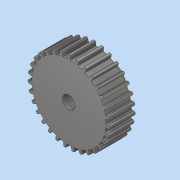
# Autodesk Inventor part: PinionGear
Saved by Autodesk Inventor 2017 (Build 210142000, 142)
## iProperties
Created: 2016-11-06
Part Number: PinionGear
Material: Stainless Steel, Brushed
Document SubType Name: Modeling
Designer: techn
Density: 8 g/cm^3
Appearance: Stainless - Brushed
Author: techn
Comments: 31 Tooth Traxxas Pinion Gear
Autodesk Inventor part; units mm, degrees
ref_plane "YZ Plane" through (0, 0, 0) normal (1, 0, 0) x (0, 1, 0)
ref_plane "XZ Plane" through (0, 0, 0) normal (0, 1, 0) x (-1, 0, 0)
ref_plane "XY Plane" through (0, 0, 0) normal (0, 0, 1) x (1, 0, 0)
sketch "Sketch1" plane through (0, 0, 0) normal (0, 0, 1) x (1, 0, 0)
  circle A0 centre (0, 0) radius 3.7465
  dimension "d0" = 7.493
  constraints: 1 centre point, 1 coincident
  measures "d0" diameter of A0
extrude "Extrusion1" add sketch "Sketch1" along normal blind 10.5156
sketch "Sketch2" plane through (0, 0, 10.5156) normal (0, 0, 1) x (1, 0, 0)
  circle A0 centre (0, 0) radius 10.16
  dimension "d3" = 20.32
  constraints: 1 centre point, 1 coincident
  measures "d3" diameter of A0
extrude "Extrusion2" add sketch "Sketch2" against normal blind 6.35
sketch "Sketch4" plane through (0, 0, 10.5156) normal (0, 0, 1) x (1, 0, 0)
  circle A0 centre (0, 0) radius 1.5875
  dimension "d6" = 3.175
  constraints: 1 centre point, 1 coincident
  measures "d6" diameter of A0
extrude "Extrusion3" cut sketch "Sketch4" against normal through all
sketch "Sketch5" plane through (0, 0, 10.5156) normal (0, 0, 1) x (1, 0, 0)
  circle A0 centre (0, 0) radius 9.2075
  line L0 (0.3683, 9.2001) -> (0.3683, 9.7081)
  line L1 (0.3683, 9.7081) -> (0.2667, 10.16)
  line L2 (0.2667, 10.16) -> (-0.2667, 10.16)
  line L3 (-0.2667, 10.16) -> (-0.3683, 9.7081)
  line L4 (-0.3683, 9.7081) -> (-0.3683, 9.2001)
  line L5 (-0.3683, 9.2001) -> (0.3683, 9.2001)
  line L6 (-2.315, 9.4353) -> (-2.2127, 8.9377)
  line L7 (-2.3064, 9.8983) -> (-2.315, 9.4353)
  line L8 (-1.784, 10.0057) -> (-2.3064, 9.8983)
  line L9 (-1.5935, 9.5835) -> (-1.784, 10.0057)
  line L10 (-1.4912, 9.0859) -> (-1.5935, 9.5835)
  line L11 (-2.2127, 8.9377) -> (-1.4912, 9.0859)
  line L12 (-4.1669, 8.7761) -> (-3.9666, 8.3093)
  line L13 (-4.2517, 9.2314) -> (-4.1669, 8.7761)
  line L14 (-3.7616, 9.4418) -> (-4.2517, 9.2314)
  line L15 (-3.49, 9.0666) -> (-3.7616, 9.4418)
  line L16 (-3.2897, 8.5998) -> (-3.49, 9.0666)
  line L17 (-3.9666, 8.3093) -> (-3.2897, 8.5998)
  line L18 (-5.8482, 7.7577) -> (-5.558, 7.3407)
  line L19 (-6.023, 8.1866) -> (-5.8482, 7.7577)
  line L20 (-5.5852, 8.4913) -> (-6.023, 8.1866)
  line L21 (-5.2437, 8.1785) -> (-5.5852, 8.4913)
  line L22 (-4.9535, 7.7615) -> (-5.2437, 8.1785)
  line L23 (-5.558, 7.3407) -> (-4.9535, 7.7615)
  line L24 (-7.2901, 6.4216) -> (-6.9219, 6.0716)
  line L25 (-7.5476, 6.8066) -> (-7.2901, 6.4216)
  line L26 (-7.1801, 7.1932) -> (-7.5476, 6.8066)
  line L27 (-6.7826, 6.9555) -> (-7.1801, 7.1932)
  line L28 (-6.4144, 6.6055) -> (-6.7826, 6.9555)
  line L29 (-6.9219, 6.0716) -> (-6.4144, 6.6055)
  line L30 (-8.4336, 4.8227) -> (-8.0025, 4.554)
  line L31 (-8.7633, 5.1479) -> (-8.4336, 4.8227)
  line L32 (-8.4812, 5.6006) -> (-8.7633, 5.1479)
  line L33 (-8.0439, 5.4478) -> (-8.4812, 5.6006)
  line L34 (-7.6128, 5.1791) -> (-8.0439, 5.4478)
  line L35 (-8.0025, 4.554) -> (-7.6128, 5.1791)
  line L36 (-9.2317, 3.0263) -> (-8.7554, 2.8499)
  line L37 (-9.6202, 3.2785) -> (-9.2317, 3.0263)
  line L38 (-9.4349, 3.7787) -> (-9.6202, 3.2785)
  line L39 (-8.9759, 3.7171) -> (-9.4349, 3.7787)
  line L40 (-8.4995, 3.5406) -> (-8.9759, 3.7171)
  line L41 (-8.7554, 2.8499) -> (-8.4995, 3.5406)
  line L42 (-9.652, 1.106) -> (-9.1498, 1.0291)
  line L43 (-10.0832, 1.2749) -> (-9.652, 1.106)
  line L44 (-10.0025, 1.8021) -> (-10.0832, 1.2749)
  line L45 (-9.5404, 1.8341) -> (-10.0025, 1.8021)
  line L46 (-9.0383, 1.7572) -> (-9.5404, 1.8341)
  line L47 (-9.1498, 1.0291) -> (-9.0383, 1.7572)
  line L48 (-9.677, -0.8595) -> (-9.1697, -0.8338)
  line L49 (-10.1335, -0.781) -> (-9.677, -0.8595)
  line L50 (-10.1605, -0.2482) -> (-10.1335, -0.781)
  line L51 (-9.7143, -0.1239) -> (-10.1605, -0.2482)
  line L52 (-9.207, -0.0982) -> (-9.7143, -0.1239)
  line L53 (-9.1697, -0.8338) -> (-9.207, -0.0982)
  line L54 (-9.3059, -2.7899) -> (-8.8141, -2.6626)
  line L55 (-9.7688, -2.8048) -> (-9.3059, -2.7899)
  line L56 (-9.9025, -2.2884) -> (-9.7688, -2.8048)
  line L57 (-9.4905, -2.0768) -> (-9.9025, -2.2884)
  line L58 (-8.9988, -1.9495) -> (-9.4905, -2.0768)
  line L59 (-8.8141, -2.6626) -> (-8.9988, -1.9495)
  line L60 (-8.5538, -4.6061) -> (-8.0977, -4.3823)
  line L61 (-9.0042, -4.7138) -> (-8.5538, -4.6061)
  line L62 (-9.2391, -4.235) -> (-9.0042, -4.7138)
  line L63 (-8.8782, -3.9447) -> (-9.2391, -4.235)
  line L64 (-8.4221, -3.721) -> (-8.8782, -3.9447)
  line L65 (-8.0977, -4.3823) -> (-8.4221, -3.721)
  line L66 (-7.4515, -6.2336) -> (-7.0498, -5.9227)
  line L67 (-7.871, -6.4299) -> (-7.4515, -6.2336)
  line L68 (-8.1975, -6.0081) -> (-7.871, -6.4299)
  line L69 (-7.9024, -5.6512) -> (-8.1975, -6.0081)
  line L70 (-7.5007, -5.3402) -> (-7.9024, -5.6512)
  line L71 (-7.0498, -5.9227) -> (-7.5007, -5.3402)
  line L72 (-6.0442, -7.606) -> (-5.7133, -7.2206)
  line L73 (-6.4156, -7.8827) -> (-6.0442, -7.606)
  line L74 (-6.8203, -7.5353) -> (-6.4156, -7.8827)
  line L75 (-6.6031, -7.1262) -> (-6.8203, -7.5353)
  line L76 (-6.2722, -6.7408) -> (-6.6031, -7.1262)
  line L77 (-5.7133, -7.2206) -> (-6.2722, -6.7408)
  line L78 (-4.3894, -8.667) -> (-4.1428, -8.2228)
  line L79 (-4.6975, -9.0128) -> (-4.3894, -8.667)
  line L80 (-5.1639, -8.7539) -> (-4.6975, -9.0128)
  line L81 (-5.0334, -8.3095) -> (-5.1639, -8.7539)
  line L82 (-4.7869, -7.8654) -> (-5.0334, -8.3095)
  line L83 (-4.1428, -8.2228) -> (-4.7869, -7.8654)
  line L84 (-2.5548, -9.3732) -> (-2.4028, -8.8885)
  line L85 (-2.7871, -9.7739) -> (-2.5548, -9.3732)
  line L86 (-3.296, -9.6142) -> (-2.7871, -9.7739)
  line L87 (-3.2577, -9.1527) -> (-3.296, -9.6142)
  line L88 (-3.1056, -8.668) -> (-3.2577, -9.1527)
  line L89 (-2.4028, -8.8885) -> (-3.1056, -8.668)
  line L90 (-0.6157, -9.6956) -> (-0.5644, -9.1902)
  line L91 (-0.7625, -10.1349) -> (-0.6157, -9.6956)
  line L92 (-1.2932, -10.0809) -> (-0.7625, -10.1349)
  line L93 (-1.3486, -9.6211) -> (-1.2932, -10.0809)
  line L94 (-1.2972, -9.1157) -> (-1.3486, -9.6211)
  line L95 (-0.5644, -9.1902) -> (-1.2972, -9.1157)
  line L96 (1.3486, -9.6211) -> (1.2972, -9.1157)
  line L97 (1.2932, -10.0809) -> (1.3486, -9.6211)
  line L98 (0.7625, -10.1349) -> (1.2932, -10.0809)
  line L99 (0.6157, -9.6956) -> (0.7625, -10.1349)
  line L100 (0.5644, -9.1902) -> (0.6157, -9.6956)
  line L101 (1.2972, -9.1157) -> (0.5644, -9.1902)
  line L102 (3.2577, -9.1527) -> (3.1056, -8.668)
  line L103 (3.296, -9.6142) -> (3.2577, -9.1527)
  line L104 (2.7871, -9.7739) -> (3.296, -9.6142)
  line L105 (2.5548, -9.3732) -> (2.7871, -9.7739)
  line L106 (2.4028, -8.8885) -> (2.5548, -9.3732)
  line L107 (3.1056, -8.668) -> (2.4028, -8.8885)
  line L108 (5.0334, -8.3095) -> (4.7869, -7.8654)
  line L109 (5.1639, -8.7539) -> (5.0334, -8.3095)
  line L110 (4.6975, -9.0128) -> (5.1639, -8.7539)
  line L111 (4.3894, -8.667) -> (4.6975, -9.0128)
  line L112 (4.1428, -8.2228) -> (4.3894, -8.667)
  line L113 (4.7869, -7.8654) -> (4.1428, -8.2228)
  line L114 (6.6031, -7.1262) -> (6.2722, -6.7408)
  line L115 (6.8203, -7.5353) -> (6.6031, -7.1262)
  line L116 (6.4156, -7.8827) -> (6.8203, -7.5353)
  line L117 (6.0442, -7.606) -> (6.4156, -7.8827)
  line L118 (5.7133, -7.2206) -> (6.0442, -7.606)
  line L119 (6.2722, -6.7408) -> (5.7133, -7.2206)
  line L120 (7.9024, -5.6512) -> (7.5007, -5.3402)
  line L121 (8.1975, -6.0081) -> (7.9024, -5.6512)
  line L122 (7.871, -6.4299) -> (8.1975, -6.0081)
  line L123 (7.4515, -6.2336) -> (7.871, -6.4299)
  line L124 (7.0498, -5.9227) -> (7.4515, -6.2336)
  line L125 (7.5007, -5.3402) -> (7.0498, -5.9227)
  line L126 (8.8782, -3.9447) -> (8.4221, -3.721)
  line L127 (9.2391, -4.235) -> (8.8782, -3.9447)
  line L128 (9.0042, -4.7138) -> (9.2391, -4.235)
  line L129 (8.5538, -4.6061) -> (9.0042, -4.7138)
  line L130 (8.0977, -4.3823) -> (8.5538, -4.6061)
  line L131 (8.4221, -3.721) -> (8.0977, -4.3823)
  line L132 (9.4905, -2.0768) -> (8.9988, -1.9495)
  line L133 (9.9025, -2.2884) -> (9.4905, -2.0768)
  line L134 (9.7688, -2.8048) -> (9.9025, -2.2884)
  line L135 (9.3059, -2.7899) -> (9.7688, -2.8048)
  line L136 (8.8141, -2.6626) -> (9.3059, -2.7899)
  line L137 (8.9988, -1.9495) -> (8.8141, -2.6626)
  line L138 (9.7143, -0.1239) -> (9.207, -0.0982)
  line L139 (10.1605, -0.2482) -> (9.7143, -0.1239)
  line L140 (10.1335, -0.781) -> (10.1605, -0.2482)
  line L141 (9.677, -0.8595) -> (10.1335, -0.781)
  line L142 (9.1697, -0.8338) -> (9.677, -0.8595)
  line L143 (9.207, -0.0982) -> (9.1697, -0.8338)
  line L144 (9.5404, 1.8341) -> (9.0383, 1.7572)
  line L145 (10.0025, 1.8021) -> (9.5404, 1.8341)
  line L146 (10.0832, 1.2749) -> (10.0025, 1.8021)
  line L147 (9.652, 1.106) -> (10.0832, 1.2749)
  line L148 (9.1498, 1.0291) -> (9.652, 1.106)
  line L149 (9.0383, 1.7572) -> (9.1498, 1.0291)
  line L150 (8.9759, 3.7171) -> (8.4995, 3.5406)
  line L151 (9.4349, 3.7787) -> (8.9759, 3.7171)
  line L152 (9.6202, 3.2785) -> (9.4349, 3.7787)
  line L153 (9.2317, 3.0263) -> (9.6202, 3.2785)
  line L154 (8.7554, 2.8499) -> (9.2317, 3.0263)
  line L155 (8.4995, 3.5406) -> (8.7554, 2.8499)
  line L156 (8.0439, 5.4478) -> (7.6128, 5.1791)
  line L157 (8.4812, 5.6006) -> (8.0439, 5.4478)
  line L158 (8.7633, 5.1479) -> (8.4812, 5.6006)
  line L159 (8.4336, 4.8227) -> (8.7633, 5.1479)
  line L160 (8.0025, 4.554) -> (8.4336, 4.8227)
  line L161 (7.6128, 5.1791) -> (8.0025, 4.554)
  line L162 (6.7826, 6.9555) -> (6.4144, 6.6055)
  line L163 (7.1801, 7.1932) -> (6.7826, 6.9555)
  line L164 (7.5476, 6.8066) -> (7.1801, 7.1932)
  line L165 (7.2901, 6.4216) -> (7.5476, 6.8066)
  line L166 (6.9219, 6.0716) -> (7.2901, 6.4216)
  line L167 (6.4144, 6.6055) -> (6.9219, 6.0716)
  line L168 (5.2437, 8.1785) -> (4.9535, 7.7615)
  line L169 (5.5852, 8.4913) -> (5.2437, 8.1785)
  line L170 (6.023, 8.1866) -> (5.5852, 8.4913)
  line L171 (5.8482, 7.7577) -> (6.023, 8.1866)
  line L172 (5.558, 7.3407) -> (5.8482, 7.7577)
  line L173 (4.9535, 7.7615) -> (5.558, 7.3407)
  line L174 (3.49, 9.0666) -> (3.2897, 8.5998)
  line L175 (3.7616, 9.4418) -> (3.49, 9.0666)
  line L176 (4.2517, 9.2314) -> (3.7616, 9.4418)
  line L177 (4.1669, 8.7761) -> (4.2517, 9.2314)
  line L178 (3.9666, 8.3093) -> (4.1669, 8.7761)
  line L179 (3.2897, 8.5998) -> (3.9666, 8.3093)
  line L180 (1.5935, 9.5835) -> (1.4912, 9.0859)
  line L181 (1.784, 10.0057) -> (1.5935, 9.5835)
  line L182 (2.3064, 9.8983) -> (1.784, 10.0057)
  line L183 (2.315, 9.4353) -> (2.3064, 9.8983)
  line L184 (2.2127, 8.9377) -> (2.315, 9.4353)
  line L185 (1.4912, 9.0859) -> (2.2127, 8.9377)
  circle A1 centre (0, 0) radius 11.1454
  dimension "d9" = 18.415
  dimension "d12" = 360
  dimension "d14" = 0.508
  dimension "d15" = 0.5334
  dimension "d16" = 0.7366
  dimension "d17" = 0.9599
  dimension "d18" = 10.16
  constraints: 372 end point, 2 centre point, 2 coincident, 2 equal length, 2 horizontal, 2 point on circle, 1 perpendicular, 1 vertical, 373 other
  measures "d9" diameter of A0
  measures "d14" distance of L0.start L0.end
  measures "d15" distance of L1.end L2.end
  measures "d16" distance of L4.end L0.start
  measures "d17" distance between parallel lines of L2 L5
  measures "d18" distance from line of point (0, 0) L2
extrude "Extrusion4" cut sketch "Sketch5" against normal up to surface (6.35 mm away)
body "Solid1"
